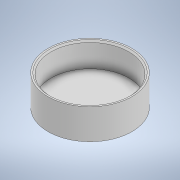
# Autodesk Inventor part: TubeCap
Saved by Autodesk Inventor 2020 (Build 240168000, 168)
## iProperties
Created: 2020-06-10
Part Number: TubeCap
Material: Generic
Document SubType Name: Modeling
Designer: antho
Density: 1 g/cm^3
Appearance: Default
Author: antho
Autodesk Inventor part; units mm, degrees
ref_plane "YZ Plane" through (0, 0, 0) normal (1, 0, 0) x (0, 1, 0)
ref_plane "XZ Plane" through (0, 0, 0) normal (0, 1, 0) x (-1, 0, 0)
ref_plane "XY Plane" through (0, 0, 0) normal (0, 0, 1) x (1, 0, 0)
sketch "Sketch1" plane through (0, 0, 0) normal (0, 1, 0) x (-1, 0, 0)
  circle A0 centre (0, 0) radius 12.825
  circle A1 centre (0, 0) radius 13.825
  dimension "d0" = 25.65
  dimension "d1" = 27.65
  constraints: 2 centre point, 2 coincident
  measures "d0" diameter of A0
  measures "d1" diameter of A1
extrude "Extrusion1" add sketch "Sketch1" along normal blind 10 contours A0 | A1
sketch "Sketch3" plane through (0, 10, 0) normal (0, 1, 0) x (1, 0, 0)
  circle A0 centre (0, 0) radius 12.825
  circle A1 centre (0, 0) radius 13.825
  dimension "d11" = 25.65
  dimension "d12" = 27.65
  constraints: 2 centre point, 2 coincident
  measures "d11" diameter of A0
  measures "d12" diameter of A1
extrude "Extrusion3" cut sketch "Sketch3" against normal blind 8 contours A0
chamfer "Chamfer2" distance 0.5 angle 45 1 edges at (-12.825, 10, 0)
body "Solid1"
